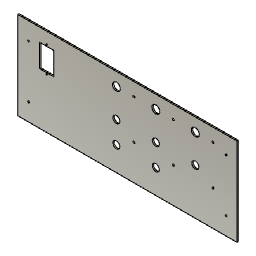
Control box rear (Autodesk Fusion 360 design; units mm, degrees)
Autodesk Fusion 360 part; units mm, degrees
sketch "Panel" plane through (0, 0, 0) normal (0, 1, 0) x (1, 0, 0)
  line L0 (-250, -13) -> (250, -13)
  line L1 (250, -13) -> (250, -213)
  line L2 (250, -213) -> (-250, -213)
  line L3 (-250, -213) -> (-250, -13)
  line L4 (-200, -183) -> (-168, -183)
  line L5 (-168, -183) -> (-168, -131)
  line L6 (-168, -131) -> (-200, -131)
  line L7 (-200, -131) -> (-200, -183)
  line L8 (-184, -114.7229) -> (-184, -199.089) construction
  circle A0 centre (-184, -186.25) radius 1.75
  circle A1 centre (-184, -127.75) radius 1.75
  line L9 (-200, -157) -> (-168, -157) construction
  line L10 (-225, -213) -> (-225, -13) construction
  circle A2 centre (-225, -53) radius 2
  circle A3 centre (-225, -173) radius 2
  line L11 (225, -213) -> (225, -209.3492) construction
  line L12 (225, -209.3492) -> (225, -13) construction
  circle A4 centre (225, -53) radius 2
  circle A5 centre (225, -173) radius 2
  line L13 (220.184, -168) -> (-130.7385, -168) construction
  line L14 (220.184, -183) -> (-130.7385, -183) construction
  line L15 (220.184, -118) -> (-123.7941, -118) construction
  line L16 (220.184, -93) -> (-123.7941, -93) construction
  line L17 (220.184, -68) -> (-123.7941, -68) construction
  line L18 (195, -213) -> (195, -38) construction
  line L19 (105, -213) -> (105, -38) construction
  line L20 (15, -213) -> (15, -38) construction
  circle A6 centre (195, -183) radius 2.25
  circle A7 centre (195, -93) radius 2.25
  circle A8 centre (105, -93) radius 2.25
  circle A9 centre (105, -183) radius 2.25
  circle A10 centre (15, -183) radius 2.25
  circle A11 centre (15, -93) radius 2.25
  line L21 (155, -183) -> (155, -68) construction
  line L22 (65, -183) -> (65, -68) construction
  line L23 (-25, -183) -> (-25, -68) construction
  circle A12 centre (155, -183) radius 9
  circle A13 centre (65, -183) radius 9
  circle A14 centre (-25, -183) radius 9
  circle A15 centre (155, -118) radius 8
  circle A16 centre (65, -118) radius 8
  circle A17 centre (-25, -118) radius 8
  circle A18 centre (65, -68) radius 8
  circle A19 centre (-25, -68) radius 8
  dimension "d1" = 500
  dimension "d2" = 200
  dimension "d3" = 13
  dimension "d4" = 250
  dimension "d5" = 32
  dimension "d6" = 52
  dimension "d7" = 50
  dimension "d8" = 30
  dimension "d9" = 3.5
  dimension "d10" = 3.5
  dimension "d11" = 29.25
  dimension "d12" = 29.25
  dimension "d13" = 25
  dimension "d14" = 4
  dimension "d15" = 4
  dimension "d16" = 25
  dimension "d17" = 4
  dimension "d18" = 4
  dimension "d19" = 40
  dimension "d20" = 40
  dimension "d21" = 40
  dimension "d22" = 40
  dimension "d23" = 45
  dimension "d24" = 30
  dimension "d25" = 95
  dimension "d26" = 90
  dimension "d27" = 50
  dimension "d29" = 55
  dimension "d30" = 90
  dimension "d31" = 90
  dimension "d35" = 4.5
  dimension "d36" = 4.5
  dimension "d37" = 4.5
  dimension "d38" = 4.5
  dimension "d39" = 4.5
  dimension "d40" = 4.5
  dimension "d44" = 40
  dimension "d45" = 40
  dimension "d46" = 40
  dimension "d47" = 18
  dimension "d48" = 18
  dimension "d49" = 18
  dimension "d50" = 16
  dimension "d51" = 16
  dimension "d52" = 16
  dimension "d53" = 16
  dimension "d54" = 16
  constraint horizontal L0
  constraint vertical L1
  constraint horizontal L2
  constraint vertical L3
  constraint horizontal L4
  constraint vertical L5
  constraint horizontal L6
  constraint vertical L7
  constraint perpendicular L4 L8
  constraint coincident L8 A0.centre
  constraint coincident L8 A1.centre
  constraint midpoint L7 L9.start
  constraint midpoint L5 L9.end
  constraint coincident L2 L10.start
  constraint coincident L0 L10.end
  constraint perpendicular L0 L10
  constraint coincident L10 A2.centre
  constraint coincident L10 A3.centre
  constraint coincident L2 L11.start
  constraint perpendicular L2 L11
  constraint coincident L0 L12.end
  constraint perpendicular L0 L12
  constraint coincident L12 A4.centre
  constraint coincident L12 A5.centre
  constraint perpendicular L12 L13
  constraint perpendicular L12 L14
  constraint perpendicular L12 L15
  constraint perpendicular L12 L16
  constraint perpendicular L12 L17
  constraint coincident L2 L18.start
  constraint perpendicular L17 L18
  constraint coincident L2 L19.start
  constraint perpendicular L17 L19
  constraint coincident L2 L20.start
  constraint perpendicular L16 L20
  constraint coincident L14 A6.centre
  constraint coincident L18 A6.centre
  constraint coincident L16 A7.centre
  constraint coincident L18 A7.centre
  constraint coincident L16 A8.centre
  constraint coincident L19 A8.centre
  constraint coincident L19 A9.centre
  constraint coincident L14 A9.centre
  constraint coincident L14 A10.centre
  constraint coincident L20 A10.centre
  constraint coincident L20 A11.centre
  constraint coincident L16 A11.centre
  constraint coincident L14 L21.start
  constraint coincident L17 L21.end
  constraint perpendicular L17 L21
  constraint coincident L14 L22.start
  constraint coincident L17 L22.end
  constraint perpendicular L17 L22
  constraint coincident L14 L23.start
  constraint coincident L17 L23.end
  constraint perpendicular L17 L23
  constraint coincident L21.start A12.centre
  constraint coincident L22.start A13.centre
  constraint coincident L23.start A14.centre
  constraint coincident L21 A15.centre
  constraint coincident L15 A15.centre
  constraint coincident L15 A16.centre
  constraint coincident L22 A16.centre
  constraint coincident L15 A17.centre
  constraint coincident L23 A17.centre
  constraint coincident L22.end A18.centre
  constraint coincident L23.end A19.centre
  measures "d1" distance of L0.start L0.end
  measures "d2" distance of L0.start L2.end
  measures "d3" distance of origin L0
  measures "d4" distance of origin L3
  measures "d5" distance of L4.start L4.end
  measures "d6" distance of L4.start L6.end
  measures "d7" distance of L3 L7
  measures "d8" distance of L2 L4
  measures "d9" diameter of A0
  measures "d10" diameter of A1
  measures "d11" distance of A0.centre L9
  measures "d12" distance of A1.centre L9
  measures "d13" distance of L3 L10
  measures "d14" diameter of A2
  measures "d15" diameter of A3
  measures "d16" distance of L1 L12
  measures "d17" diameter of A4
  measures "d18" diameter of A5
  measures "d19" distance of L0 A2.centre
  measures "d20" distance of L2 A3.centre
  measures "d21" distance of L2 A5.centre
  measures "d22" distance of L0 A4.centre
  measures "d23" distance of L2 L13
  measures "d24" distance of L2 L14
  measures "d25" distance of L2 L15
  measures "d26" distance of L14 L16
  measures "d27" distance of L15 L17
  measures "d29" distance of L1 L18
  measures "d30" distance of L18 L19
  measures "d31" distance of L19 L20
  measures "d35" diameter of A6
  measures "d36" diameter of A7
  measures "d37" diameter of A8
  measures "d38" diameter of A9
  measures "d39" diameter of A10
  measures "d40" diameter of A11
  measures "d44" distance of L20 L23
  measures "d45" distance of L18 L21
  measures "d46" distance of L19 L22
  measures "d47" diameter of A12
  measures "d48" diameter of A13
  measures "d49" diameter of A14
  measures "d50" diameter of A15
  measures "d51" diameter of A16
  measures "d52" diameter of A17
  measures "d53" diameter of A18
  measures "d54" diameter of A19
extrude "Extrude1" add sketch "Panel" along normal blind 3
equation "d4 = d1 / 2"
equation "d12 = d11"
equation "d15 = d14"
equation "d16 = d13"
equation "d17 = d14"
equation "d18 = d14"
equation "d20 = d19"
equation "d21 = d19"
equation "d22 = d19"
equation "d31 = d30"
equation "d36 = d35"
equation "d37 = d35"
equation "d38 = d35"
equation "d39 = d35"
equation "d40 = d35"
equation "d45 = d44"
equation "d46 = d44"
equation "d48 = d47"
equation "d49 = d47"
equation "d51 = d50"
equation "d52 = d50"
equation "d53 = d50"
equation "d54 = d50"
named bodies: "Panel"
